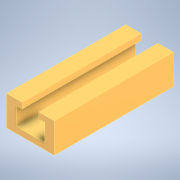
# Autodesk Inventor part: jeep pvc connector
Saved by Autodesk Inventor 2021 (Build 250183000, 183)
## iProperties
Created: 2020-07-11
Part Number: jeep pvc connector
Material: Generic
Document SubType Name: Modeling
Designer: Shannon
Density: 1 g/cm^3
Appearance: Gold
Author: Shannon
Autodesk Inventor part; units mm, degrees
ref_plane "YZ Plane" through (0, 0, 0) normal (1, 0, 0) x (0, 1, 0)
ref_plane "XZ Plane" through (0, 0, 0) normal (0, 1, 0) x (-1, 0, 0)
ref_plane "XY Plane" through (0, 0, 0) normal (0, 0, 1) x (1, 0, 0)
sketch "Sketch1" plane through (0, 0, 0) normal (0, 1, 0) x (-1, 0, 0)
  line L0 (0, 52.8555) -> (50.8, 52.8555)
  line L1 (50.8, 52.8555) -> (50.8, -74.1445)
  line L2 (50.8, -74.1445) -> (0, -74.1445)
  line L3 (0, -74.1445) -> (0, 52.8555)
  point P0 (0, 0)
  dimension "d0" = 50.8
  dimension "d1" = 127
  constraints: 8 end point, 2 parallel, 1 horizontal, 1 perpendicular
  measures "d0" distance of L0.start L0.end
  measures "d1" distance of L0.end L1.end
extrude "Extrusion1" add sketch "Sketch1" along normal blind 6.35
sketch "Sketch2" plane through (0, 6.35, 0) normal (0, 1, 0) x (1, 0, 0)
  line L0 (-50.8, -52.8555) -> (0, -52.8555) projected
  line L1 (0, 74.1445) -> (-50.8, 74.1445) projected
  line L2 (0, -52.8555) -> (-10.16, -52.8555)
  line L3 (-10.16, -52.8555) -> (-10.16, 74.1445)
  line L4 (-10.16, 74.1445) -> (0, 74.1445)
  line L5 (0, 74.1445) -> (0, -52.8555)
  line L6 (-50.8, 74.1445) -> (-40.64, 74.1445)
  line L7 (-40.64, 74.1445) -> (-40.64, -52.8555)
  line L8 (-40.64, -52.8555) -> (-50.8, -52.8555)
  line L9 (-50.8, -52.8555) -> (-50.8, 74.1445)
  point P0 (0, 0)
  point P1 (-40.64, -52.8555)
  dimension "d4" = 10.16
  dimension "d5" = 10.16
  constraints: 16 end point, 4 parallel, 2 horizontal, 2 perpendicular, 2 point on line
  measures "d4" distance between parallel lines of L9 L7
  measures "d5" distance between parallel lines of L5 L3
extrude "Extrusion2" add sketch "Sketch2" along normal blind 25.4 contours L9 L1 L7 L0 | L3 L1 L5 L0
sketch "Sketch3" plane through (-40.64, 6.35, 52.8555) normal (1, 0, 0) x (0, 0, -1)
  line L0 (127, 25.4) -> (0, 25.4) projected
  line L1 (0, 25.4) -> (127, 25.4)
  line L2 (127, 25.4) -> (127, 19.05)
  line L3 (127, 19.05) -> (0, 19.05)
  line L4 (0, 19.05) -> (0, 25.4)
  point P0 (52.8555, -6.35)
  dimension "d8" = 6.35
  constraints: 8 end point, 2 parallel, 1 horizontal, 1 perpendicular
  measures "d8" distance between parallel lines of L3 L0
extrude "Extrusion3" add sketch "Sketch3" along normal blind 6.35
sketch "Sketch4" plane through (-10.16, 6.35, -74.1445) normal (-1, 0, 0) x (0, 0, 1)
  line L0 (0, 25.4) -> (127, 25.4) projected
  line L1 (127, 25.4) -> (127, 19.05) projected
  line L2 (0, 25.4) -> (127, 25.4)
  line L3 (127, 25.4) -> (127, 19.05)
  line L4 (127, 19.05) -> (0, 19.05)
  line L5 (0, 19.05) -> (0, 25.4)
  point P0 (74.1445, -6.35)
  constraints: 8 end point, 2 parallel, 1 horizontal, 1 perpendicular
extrude "Extrusion4" add sketch "Sketch4" along normal blind 6.35
sketch "Sketch5" plane through (0, 0, 0) normal (0, -1, 0) x (1, 0, 0)
  circle A0 centre (-25.4, -10.6445) radius 8.729
  line L0 (0, 52.8555) -> (0, -74.1445) projected
  line L1 (0, -74.1445) -> (-50.8, -74.1445) projected
  point P0 (0, 0)
  dimension "d13" = 25.4
  dimension "d14" = 63.5
  constraints: 1 centre point
  measures "d13" distance from line of L0 A0.centre
  measures "d14" distance from line of L1 A0.centre
extrude "Extrusion5" cut sketch "Sketch5" against normal up to surface (6.35 mm away)
body "Solid1"
